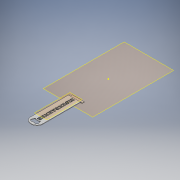
# Autodesk Inventor part: Rost_Heber
Saved by Autodesk Inventor 2018 (Build 220112000, 112)
## iProperties
Created: 2017-10-08
Part Number: Rost_Heber
Material: Generisch
Document SubType Name: Blech
Designer: Jan
Density: 1 g/cm^3
Sheet Metal Rule: Standard_mm
Appearance: Vorgabe
Flat Pattern Width: 4.3 cm
Flat Pattern Length: 17.3098 cm
Flat Pattern Area: 74.432 cm^2
Sheet Metal Width: 43,000 mm
Sheet Metal Length: 173,098 mm
Sheet Metal Area: 7443,205 mm^2
Author: Jan
Autodesk Inventor part; units mm, degrees
ref_plane "YZ Plane" through (0, 0, 0) normal (1, 0, 0) x (0, 1, 0)
ref_plane "XZ Plane" through (0, 0, 0) normal (0, 1, 0) x (-1, 0, 0)
ref_plane "XY Plane" through (0, 0, 0) normal (0, 0, 1) x (1, 0, 0)
ref_plane "Arbeitsebene1" through (0, 0, 0) normal (0, 0, 1) x (1, 0, 0)
sketch "Skizze1" plane through (0, 0, 0) normal (0, 0, 1) x (1, 0, 0)
  arc A0 (31.5, -113.5) -> (26.5, -108.5) centre (26.5, -113.5) ccw
  line L0 (26.5, -108.5) -> (-26.5, -108.5)
  arc A1 (-26.5, -108.5) -> (-31.5, -113.5) centre (-26.5, -113.5) ccw
  line L1 (-31.5, -113.5) -> (-31.5, -124.5)
  line L2 (-31.5, -124.5) -> (-71, -124.5)
  arc A2 (-73, -122.5) -> (-71, -124.5) centre (-71, -122.5) ccw
  line L3 (-73, -122.5) -> (-73, 122.5)
  arc A3 (-71, 124.5) -> (-73, 122.5) centre (-71, 122.5) ccw
  line L4 (-71, 124.5) -> (71, 124.5)
  arc A4 (73, 122.5) -> (71, 124.5) centre (71, 122.5) ccw
  line L5 (73, 122.5) -> (73, -122.5)
  arc A5 (71, -124.5) -> (73, -122.5) centre (71, -122.5) ccw
  line L6 (71, -124.5) -> (31.5, -124.5)
  line L7 (31.5, -124.5) -> (31.5, -113.5)
  line L8 (-22.5, -122.5) -> (-22.5, -117.5)
  line L9 (-22.5, -117.5) -> (22.5, -117.5)
  line L10 (22.5, -117.5) -> (22.5, -122.5)
  line L11 (22.5, -122.5) -> (-22.5, -122.5)
  arc A6 (-81, -122.5) -> (-71, -132.5) centre (-71, -122.5) ccw
  line L12 (71, -132.5) -> (-71, -132.5)
  arc A7 (71, -132.5) -> (81, -122.5) centre (71, -122.5) ccw
  line L13 (81, 122.5) -> (81, -122.5)
  arc A8 (81, 122.5) -> (71, 132.5) centre (71, 122.5) ccw
  line L14 (-71, 132.5) -> (71, 132.5)
  arc A9 (-71, 132.5) -> (-81, 122.5) centre (-71, 122.5) ccw
  line L15 (-81, -122.5) -> (-81, 122.5)
  line L16 (-21.5, -118.5) -> (21.5, -118.5)
  line L17 (21.5, -118.5) -> (21.5, -258.5)
  line L18 (1.5, -278.5) -> (-1.5, -278.5)
  line L19 (-21.5, -258.5) -> (-21.5, -118.5)
  line L20 (-116.2995, 0) -> (116.2995, 0)
  line L21 (0, -314.1009) -> (0, 209.3497)
  arc A10 (-21.5, -258.5) -> (-1.5, -278.5) centre (-1.5, -258.5) ccw
  arc A11 (1.5, -278.5) -> (21.5, -258.5) centre (1.5, -258.5) ccw
  point P0 (0, 0)
  dimension "HeberBreite" = 43
  dimension "d3" = 1
  dimension "HeberLänge" = 160
  dimension "d5" = 20
  measures "HeberBreite" distance of L16.start L16.end
  measures "d3" distance between parallel lines of L9 L16
  measures "HeberLänge" distance between parallel lines of L18 L16
  measures "d5" radius of A10
extrude "Grobblech1" add sketch "Skizze1" along normal blind 2 contours L21 L11 L19 L16 | L16 L17 L11 L21 | L21 L12 L19 L11 | L11 L17 L12 L21 | L21 L18 A10 L19 L12 | L12 L17 A11 L18 L21
sketch "Skizze2" plane through (21.5, -120.5, 2) normal (0, 1, 0) x (-1, 0, 0)
  line L0 (43, 0) -> (0, 0)
  line L1 (0, 0) -> (0, -8.05)
  line L2 (0, -8.05) -> (43, -8.05)
  line L3 (43, -8.05) -> (43, 0)
  constraints: 6 end point, 1 horizontal, 1 perpendicular, 1 vertical
edge flange "Lasche1" height 8.05 angle 90 thickness 2 bend radius 2 thickness toward (0, 1, 0) relief tear relief width 2 relief depth 1 edges at (0, -118.5, 0) wall of the first edge with corners at (-21.5, -120.5, 2) (21.5, -120.5, 2) (21.5, -120.5, -6.05) (-21.5, -120.5, -6.05)
bend "Biegung1"
corner "Ecke1"
sketch "Skizze3" plane through (-21.5, -120.5, -4.05) normal (0, 0, -1) x (-1, 0, 0)
  line L0 (-43, 0) -> (0, 0)
  line L1 (0, 0) -> (0, 12)
  line L2 (0, 12) -> (-43, 12)
  line L3 (-43, 12) -> (-43, 0)
  constraints: 6 end point, 1 horizontal, 1 perpendicular, 1 vertical
edge flange "Lasche2" height 12 angle 90 thickness 2 bend radius 2 thickness toward (0, 0, -1) relief tear relief width 2 relief depth 1 edges at (0, -118.5, -6.05) wall of the first edge with corners at (21.5, -120.5, -4.05) (-21.5, -120.5, -4.05) (-21.5, -108.5, -4.05) (21.5, -108.5, -4.05)
bend "Biegung2"
corner "Ecke2"
sketch "Skizze5" plane through (0, 0, 2) normal (0, 0, 1) x (1, 0, 0)
  line L0 (7, -256.35) -> (7, -254.2861)
  arc A0 (10.3913, -255.0234) -> (7, -254.2861) centre (8.4432, -255.8158) ccw
  line L1 (10.3913, -255.0234) -> (13.6639, -265.2358)
  arc A1 (4.2286, -269.9021) -> (13.6639, -265.2358) centre (7.6833, -265.0153) ccw
  line L2 (21.5, -122.5) -> (-21.5, -122.5) projected
  line L3 (-21.5, -258.5) -> (-21.5, -122.5) projected
  arc A2 (-21.5, -258.5) -> (-1.5, -278.5) centre (-1.5, -258.5) ccw projected
  line L4 (21.5, -122.5) -> (21.5, -258.5) projected
  line L5 (7, -256.35) -> (0, -256.35)
  line L6 (4.2286, -269.9021) -> (0, -269.9021)
  arc A3 (-7, -254.2861) -> (-10.3039, -254.8354) centre (-8.4432, -255.8158) ccw
  line L7 (-10.3039, -254.8354) -> (-13.6607, -265.3108)
  arc A4 (-13.6607, -265.3108) -> (-4.2287, -269.9021) centre (-7.6833, -265.0153) ccw
  line L8 (-7, -256.35) -> (0, -256.35)
  line L9 (-4.2287, -269.9021) -> (0, -269.9021)
  line L10 (-7, -254.2861) -> (-7, -256.35)
  line L11 (0, -312.7) -> (0, 206.7)
  line L12 (1.5, -278.5) -> (-1.5, -278.5) projected
  arc A5 (1.5, -278.5) -> (21.5, -258.5) centre (1.5, -258.5) ccw projected
  constraints: 19 end point, 8 point on circle, 4 centre point, 3 parallel, 2 equal radius, 1 point on line, 1 vertical, 2 other
extrude "Ausklinkung1" cut sketch "Skizze5" against normal blind 2 contours L0 A0 L1 A1 L6 L11 L5 | L11 L9 A4 L7 A3 L10 L8
sketch "Skizze7" plane through (0, 0, 2) normal (0, 0, 1) x (1, 0, 0)
  point P0 (0, 0)
ref_plane "Arbeitsebene2" through (0, 0, 7) normal (0, 0, 1) x (1, 0, 0)
sketch "Skizze8" plane through (0, 0, 7) normal (0, 0, 1) x (1, 0, 0)
  line L0 (5.5899, -125.0888) -> (5.5899, -288.9625) construction
  line L1 (5.5899, -288.9625) -> (-5.6945, -288.9625) construction
  line L2 (-5.6945, -288.9625) -> (-5.6945, -125.0888) construction
  line L3 (-5.6945, -125.0888) -> (5.5899, -125.0888) construction
  line L4 (5.3803, -130.8766) -> (-5.1197, -130.8766)
  line L5 (-5.1197, -130.8766) -> (-5.1197, -126.775)
  line L6 (-5.1197, -126.775) -> (-5.1197, -126.5381)
  spline S0 degree 2 poles (-5.1197, -126.5381) (-5.1197, -126.2008) (-4.9101, -125.8453) (-4.7187, -125.8453) knots 0 0 0 1 2 2 2
  spline S1 degree 2 poles (-4.7187, -125.8453) (-4.4088, -125.8453) (-4.3085, -126.2099) knots 0 0 0 1 1 1
  spline S2 degree 2 poles (-4.3085, -126.2099) (-4.2174, -126.5198) (-4.1809, -126.6201) (-4.108, -126.6748) knots 0 0 0 1 2 2 2
  spline S3 degree 2 poles (-4.108, -126.6748) (-3.9895, -126.7842) (-3.7161, -126.7842) knots 0 0 0 1 1 1
  line L7 (-3.7161, -126.7842) -> (3.9766, -126.7842)
  spline S4 degree 2 poles (3.9766, -126.7842) (4.25, -126.7842) (4.3685, -126.6748) knots 0 0 0 1 1 1
  spline S5 degree 2 poles (4.3685, -126.6748) (4.4415, -126.6201) (4.4779, -126.5198) (4.5599, -126.2099) knots 0 0 0 1 2 2 2
  spline S6 degree 2 poles (4.5599, -126.2099) (4.6602, -125.8453) (4.9792, -125.8453) knots 0 0 0 1 1 1
  spline S7 degree 2 poles (4.9792, -125.8453) (5.1706, -125.8453) (5.3803, -126.2008) (5.3803, -126.5381) knots 0 0 0 1 2 2 2
  line L8 (5.3803, -126.5381) -> (5.3803, -126.775)
  line L9 (5.3803, -126.775) -> (5.3803, -130.8766)
  line L10 (-5.1197, -131.7151) -> (-4.2903, -131.7151)
  spline S8 degree 2 poles (-4.2903, -131.7151) (-4.2174, -132.3167) (-3.9348, -133.1006) (-3.6523, -133.4925) knots 0 0 0 1 2 2 2
  spline S9 degree 2 poles (-3.6523, -133.4925) (-3.3697, -133.8935) (-2.7591, -134.3584) (-2.2578, -134.5771) knots 0 0 0 1 2 2 2
  spline S10 degree 2 poles (-2.2578, -134.5771) (-2.0117, -134.6774) (-1.8385, -134.8961) (-1.8385, -135.0875) knots 0 0 0 1 2 2 2
  spline S11 degree 2 poles (-1.8385, -135.0875) (-1.8385, -135.3519) (-2.0937, -135.5524) (-2.4036, -135.5524) knots 0 0 0 1 2 2 2
  line L11 (-2.4036, -135.5524) -> (-5.1197, -135.5524)
  line L12 (-5.1197, -135.5524) -> (-5.1197, -131.7151)
  line L13 (5.3803, -131.706) -> (5.3803, -135.4248)
  line L14 (5.3803, -135.4248) -> (2.655, -135.4248)
  spline S12 degree 2 poles (2.655, -135.4248) (2.418, -135.4248) (2.2084, -135.206) (2.2084, -134.9599) knots 0 0 0 1 2 2 2
  spline S13 degree 2 poles (2.2084, -134.9599) (2.2084, -134.7594) (2.3451, -134.5771) (2.5639, -134.4951) knots 0 0 0 1 2 2 2
  spline S14 degree 2 poles (2.5639, -134.4951) (3.448, -134.1396) (4.3868, -132.7815) (4.4779, -131.706) knots 0 0 0 1 2 2 2
  line L15 (4.4779, -131.706) -> (5.3803, -131.706)
  line L16 (-0.2252, -131.6605) -> (0.668, -131.6605)
  spline S15 degree 2 poles (0.668, -131.6605) (0.8868, -132.1982) (1.3972, -132.7086) (1.8165, -132.8362) knots 0 0 0 1 2 2 2
  spline S16 degree 2 poles (1.8165, -132.8362) (2.1081, -132.9092) (2.336, -133.1461) (2.336, -133.3649) knots 0 0 0 1 2 2 2
  spline S17 degree 2 poles (2.336, -133.3649) (2.336, -133.6657) (2.1446, -133.775) knots 0 0 0 1 1 1
  spline S18 degree 2 poles (2.1446, -133.775) (2.0443, -133.8388) (1.6889, -133.8388) knots 0 0 0 1 1 1
  line L17 (1.6889, -133.8388) -> (-1.246, -133.8388)
  spline S19 degree 2 poles (-1.246, -133.8388) (-1.6106, -133.8388) (-1.8841, -133.6474) (-1.8841, -133.3831) knots 0 0 0 1 2 2 2
  spline S20 degree 2 poles (-1.8841, -133.3831) (-1.8841, -133.1735) (-1.6653, -132.9365) (-1.4101, -132.8636) knots 0 0 0 1 2 2 2
  spline S21 degree 2 poles (-1.4101, -132.8636) (-0.8815, -132.6995) (-0.3164, -132.1253) (-0.2252, -131.6605) knots 0 0 0 1 2 2 2
  line L18 (-5.1197, -141.9782) -> (-5.1197, -137.8675)
  line L19 (-5.1197, -137.8675) -> (-5.1197, -137.6305)
  spline S22 degree 2 poles (-5.1197, -137.6305) (-5.1197, -137.2933) (-4.9101, -136.9378) (-4.7187, -136.9378) knots 0 0 0 1 2 2 2
  spline S23 degree 2 poles (-4.7187, -136.9378) (-4.4088, -136.9378) (-4.3085, -137.3024) knots 0 0 0 1 1 1
  spline S24 degree 2 poles (-4.3085, -137.3024) (-4.2174, -137.6123) (-4.1809, -137.7125) (-4.108, -137.7672) knots 0 0 0 1 2 2 2
  spline S25 degree 2 poles (-4.108, -137.7672) (-3.9895, -137.8766) (-3.7161, -137.8766) knots 0 0 0 1 1 1
  line L20 (-3.7161, -137.8766) -> (3.9766, -137.8766)
  spline S26 degree 2 poles (3.9766, -137.8766) (4.25, -137.8766) (4.3685, -137.7672) knots 0 0 0 1 1 1
  spline S27 degree 2 poles (4.3685, -137.7672) (4.4415, -137.7125) (4.4779, -137.6123) (4.5599, -137.3024) knots 0 0 0 1 2 2 2
  spline S28 degree 2 poles (4.5599, -137.3024) (4.6602, -136.9378) (4.9792, -136.9378) knots 0 0 0 1 1 1
  spline S29 degree 2 poles (4.9792, -136.9378) (5.1706, -136.9378) (5.3803, -137.2933) (5.3803, -137.6305) knots 0 0 0 1 2 2 2
  line L21 (5.3803, -137.6305) -> (5.3803, -137.8675)
  line L22 (5.3803, -137.8675) -> (5.3803, -141.9782)
  line L23 (5.3803, -141.9782) -> (5.3803, -142.2151)
  spline S30 degree 2 poles (5.3803, -142.2151) (5.3803, -142.5524) (5.1706, -142.9078) (4.9792, -142.9078) knots 0 0 0 1 2 2 2
  spline S31 degree 2 poles (4.9792, -142.9078) (4.6602, -142.9078) (4.5599, -142.5433) knots 0 0 0 1 1 1
  spline S32 degree 2 poles (4.5599, -142.5433) (4.4779, -142.2334) (4.4415, -142.1331) (4.3685, -142.0784) knots 0 0 0 1 2 2 2
  spline S33 degree 2 poles (4.3685, -142.0784) (4.25, -141.969) (3.9766, -141.969) knots 0 0 0 1 1 1
  line L24 (3.9766, -141.969) -> (-3.7161, -141.969)
  spline S34 degree 2 poles (-3.7161, -141.969) (-3.9895, -141.969) (-4.108, -142.0784) knots 0 0 0 1 1 1
  spline S35 degree 2 poles (-4.108, -142.0784) (-4.1809, -142.1331) (-4.2174, -142.2334) (-4.3085, -142.5433) knots 0 0 0 1 2 2 2
  spline S36 degree 2 poles (-4.3085, -142.5433) (-4.4088, -142.9078) (-4.7187, -142.9078) knots 0 0 0 1 1 1
  spline S37 degree 2 poles (-4.7187, -142.9078) (-4.9101, -142.9078) (-5.1197, -142.5524) (-5.1197, -142.2151) knots 0 0 0 1 2 2 2
  line L25 (-5.1197, -142.2151) -> (-5.1197, -141.9782)
  line L26 (5.5899, -148.6865) -> (4.7058, -148.6865)
  spline S38 degree 2 poles (4.7058, -148.6865) (4.5691, -148.1123) (4.0222, -147.5107) (3.6303, -147.5107) knots 0 0 0 1 2 2 2
  spline S39 degree 2 poles (3.6303, -147.5107) (3.2383, -147.5107) (2.6641, -148.012) (2.3998, -148.568) knots 0 0 0 1 2 2 2
  spline S40 degree 2 poles (2.3998, -148.568) (2.2266, -148.9599) (1.7253, -150.3271) knots 0 0 0 1 1 1
  spline S41 degree 2 poles (1.7253, -150.3271) (1.4245, -151.1565) (0.9415, -152.068) (0.5769, -152.4782) knots 0 0 0 1 2 2 2
  spline S42 degree 2 poles (0.5769, -152.4782) (-0.371, -153.5628) (-1.6927, -153.5628) knots 0 0 0 1 1 1
  spline S43 degree 2 poles (-1.6927, -153.5628) (-2.677, -153.5628) (-4.3268, -152.3779) (-4.8007, -151.348) knots 0 0 0 1 2 2 2
  spline S44 degree 2 poles (-4.8007, -151.348) (-5.0468, -150.792) (-5.3294, -149.4795) (-5.3294, -148.9052) knots 0 0 0 1 2 2 2
  line L27 (-5.3294, -148.9052) -> (-4.4544, -148.9052)
  spline S45 degree 2 poles (-4.4544, -148.9052) (-4.2903, -149.7073) (-3.7161, -150.4183) (-3.2239, -150.4183) knots 0 0 0 1 2 2 2
  spline S46 degree 2 poles (-3.2239, -150.4183) (-2.7044, -150.4183) (-2.3124, -149.8623) knots 0 0 0 1 1 1
  spline S47 degree 2 poles (-2.3124, -149.8623) (-2.0572, -149.4977) (-1.6835, -148.4586) knots 0 0 0 1 1 1
  spline S48 degree 2 poles (-1.6835, -148.4586) (-1.2643, -147.3284) (-0.9088, -146.4899) (-0.6718, -146.098) knots 0 0 0 1 2 2 2
  spline S49 degree 2 poles (-0.6718, -146.098) (0.3581, -144.3662) (2.0717, -144.3662) knots 0 0 0 1 1 1
  spline S50 degree 2 poles (2.0717, -144.3662) (2.9467, -144.3662) (4.4323, -145.2321) (4.8881, -146.0068) knots 0 0 0 1 2 2 2
  spline S51 degree 2 poles (4.8881, -146.0068) (5.517, -147.0914) (5.5899, -148.6865) knots 0 0 0 1 1 1
  line L28 (-4.4544, -148.2034) -> (-5.3294, -148.2034)
  spline S52 degree 2 poles (-5.3294, -148.2034) (-5.3294, -147.4469) (-4.9739, -146.5355) knots 0 0 0 1 1 1
  spline S53 degree 2 poles (-4.9739, -146.5355) (-4.8372, -146.1891) (-4.7643, -145.9339) (-4.7643, -145.8154) knots 0 0 0 1 2 2 2
  spline S54 degree 2 poles (-4.7643, -145.8154) (-4.7643, -145.6331) (-4.8645, -145.4417) (-5.0651, -145.2412) knots 0 0 0 1 2 2 2
  spline S55 degree 2 poles (-5.0651, -145.2412) (-5.2291, -145.0771) (-5.2291, -144.8857) knots 0 0 0 1 1 1
  spline S56 degree 2 poles (-5.2291, -144.8857) (-5.2291, -144.3662) (-4.5638, -144.3662) knots 0 0 0 1 1 1
  line L29 (-4.5638, -144.3662) -> (-1.7656, -144.3662)
  spline S57 degree 2 poles (-1.7656, -144.3662) (-1.5559, -144.3662) (-1.2552, -144.6578) (-1.246, -144.8857) knots 0 0 0 1 2 2 2
  spline S58 degree 2 poles (-1.246, -144.8857) (-1.2369, -145.0862) (-1.4466, -145.3141) (-1.7109, -145.3961) knots 0 0 0 1 2 2 2
  spline S59 degree 2 poles (-1.7109, -145.3961) (-2.3671, -145.6149) (-3.5247, -146.417) (-3.9166, -146.9456) knots 0 0 0 1 2 2 2
  spline S60 degree 2 poles (-3.9166, -146.9456) (-4.3359, -147.4925) (-4.4544, -148.2034) knots 0 0 0 1 1 1
  line L30 (4.7058, -149.4157) -> (5.5534, -149.4157)
  spline S61 degree 2 poles (5.5534, -149.4157) (5.517, -149.9716) (5.3347, -150.7828) (5.0704, -151.5302) knots 0 0 0 1 2 2 2
  spline S62 degree 2 poles (5.0704, -151.5302) (5.0066, -151.7125) (5.0066, -151.831) knots 0 0 0 1 1 1
  spline S63 degree 2 poles (5.0066, -151.831) (5.0066, -152.0042) (5.1068, -152.0953) knots 0 0 0 1 1 1
  line L31 (5.1068, -152.0953) -> (5.3347, -152.2959)
  spline S64 degree 2 poles (5.3347, -152.2959) (5.5079, -152.4417) (5.5079, -152.6513) knots 0 0 0 1 1 1
  spline S65 degree 2 poles (5.5079, -152.6513) (5.5079, -152.9065) (5.2071, -153.1344) (4.8881, -153.1344) knots 0 0 0 1 2 2 2
  line L32 (4.8881, -153.1344) -> (2.3451, -153.1344)
  spline S66 degree 2 poles (2.3451, -153.1344) (2.1172, -153.1344) (1.8347, -152.8336) (1.8347, -152.5875) knots 0 0 0 1 2 2 2
  spline S67 degree 2 poles (1.8347, -152.5875) (1.8347, -152.4052) (1.9349, -152.2503) knots 0 0 0 1 1 1
  spline S68 degree 2 poles (1.9349, -152.2503) (1.9987, -152.1683) (2.1719, -152.068) (2.3816, -152.0224) knots 0 0 0 1 2 2 2
  spline S69 degree 2 poles (2.3816, -152.0224) (2.7644, -151.9131) (3.5573, -151.4209) (3.8764, -151.0836) knots 0 0 0 1 2 2 2
  spline S70 degree 2 poles (3.8764, -151.0836) (4.5053, -150.4183) (4.7058, -149.4157) knots 0 0 0 1 1 1
  line L33 (5.3803, -160.0433) -> (-5.1197, -160.0433)
  line L34 (-5.1197, -160.0433) -> (-5.1197, -155.9417)
  line L35 (-5.1197, -155.9417) -> (-5.1197, -155.7047)
  spline S71 degree 2 poles (-5.1197, -155.7047) (-5.1197, -155.3675) (-4.9101, -155.012) (-4.7187, -155.012) knots 0 0 0 1 2 2 2
  spline S72 degree 2 poles (-4.7187, -155.012) (-4.4088, -155.012) (-4.3085, -155.3766) knots 0 0 0 1 1 1
  spline S73 degree 2 poles (-4.3085, -155.3766) (-4.2174, -155.6865) (-4.1809, -155.7868) (-4.108, -155.8414) knots 0 0 0 1 2 2 2
  spline S74 degree 2 poles (-4.108, -155.8414) (-3.9895, -155.9508) (-3.7161, -155.9508) knots 0 0 0 1 1 1
  line L36 (-3.7161, -155.9508) -> (3.9766, -155.9508)
  spline S75 degree 2 poles (3.9766, -155.9508) (4.25, -155.9508) (4.3685, -155.8414) knots 0 0 0 1 1 1
  spline S76 degree 2 poles (4.3685, -155.8414) (4.4415, -155.7868) (4.4779, -155.6865) (4.5599, -155.3766) knots 0 0 0 1 2 2 2
  spline S77 degree 2 poles (4.5599, -155.3766) (4.6602, -155.012) (4.9792, -155.012) knots 0 0 0 1 1 1
  spline S78 degree 2 poles (4.9792, -155.012) (5.1706, -155.012) (5.3803, -155.3675) (5.3803, -155.7047) knots 0 0 0 1 2 2 2
  line L37 (5.3803, -155.7047) -> (5.3803, -155.9417)
  line L38 (5.3803, -155.9417) -> (5.3803, -160.0433)
  line L39 (-5.1197, -160.8818) -> (-4.2903, -160.8818)
  spline S79 degree 2 poles (-4.2903, -160.8818) (-4.2174, -161.4834) (-3.9348, -162.2672) (-3.6523, -162.6591) knots 0 0 0 1 2 2 2
  spline S80 degree 2 poles (-3.6523, -162.6591) (-3.3697, -163.0602) (-2.7591, -163.525) (-2.2578, -163.7438) knots 0 0 0 1 2 2 2
  spline S81 degree 2 poles (-2.2578, -163.7438) (-2.0117, -163.844) (-1.8385, -164.0628) (-1.8385, -164.2542) knots 0 0 0 1 2 2 2
  spline S82 degree 2 poles (-1.8385, -164.2542) (-1.8385, -164.5185) (-2.0937, -164.719) (-2.4036, -164.719) knots 0 0 0 1 2 2 2
  line L40 (-2.4036, -164.719) -> (-5.1197, -164.719)
  line L41 (-5.1197, -164.719) -> (-5.1197, -160.8818)
  line L42 (5.3803, -160.8727) -> (5.3803, -164.5914)
  line L43 (5.3803, -164.5914) -> (2.655, -164.5914)
  spline S83 degree 2 poles (2.655, -164.5914) (2.418, -164.5914) (2.2084, -164.3727) (2.2084, -164.1266) knots 0 0 0 1 2 2 2
  spline S84 degree 2 poles (2.2084, -164.1266) (2.2084, -163.9261) (2.3451, -163.7438) (2.5639, -163.6618) knots 0 0 0 1 2 2 2
  spline S85 degree 2 poles (2.5639, -163.6618) (3.448, -163.3063) (4.3868, -161.9482) (4.4779, -160.8727) knots 0 0 0 1 2 2 2
  line L44 (4.4779, -160.8727) -> (5.3803, -160.8727)
  line L45 (-0.2252, -160.8271) -> (0.668, -160.8271)
  spline S86 degree 2 poles (0.668, -160.8271) (0.8868, -161.3649) (1.3972, -161.8753) (1.8165, -162.0029) knots 0 0 0 1 2 2 2
  spline S87 degree 2 poles (1.8165, -162.0029) (2.1081, -162.0758) (2.336, -162.3128) (2.336, -162.5315) knots 0 0 0 1 2 2 2
  spline S88 degree 2 poles (2.336, -162.5315) (2.336, -162.8323) (2.1446, -162.9417) knots 0 0 0 1 1 1
  spline S89 degree 2 poles (2.1446, -162.9417) (2.0443, -163.0055) (1.6889, -163.0055) knots 0 0 0 1 1 1
  line L46 (1.6889, -163.0055) -> (-1.246, -163.0055)
  spline S90 degree 2 poles (-1.246, -163.0055) (-1.6106, -163.0055) (-1.8841, -162.8141) (-1.8841, -162.5498) knots 0 0 0 1 2 2 2
  spline S91 degree 2 poles (-1.8841, -162.5498) (-1.8841, -162.3401) (-1.6653, -162.1032) (-1.4101, -162.0302) knots 0 0 0 1 2 2 2
  spline S92 degree 2 poles (-1.4101, -162.0302) (-0.8815, -161.8662) (-0.3164, -161.292) (-0.2252, -160.8271) knots 0 0 0 1 2 2 2
  line L47 (5.3803, -171.3271) -> (-1.7291, -176.2308)
  line L48 (-1.7291, -176.2308) -> (-5.1197, -176.2308)
  line L49 (-5.1197, -176.2308) -> (-5.1197, -173.7151)
  line L50 (-5.1197, -173.7151) -> (3.8764, -167.4534)
  spline S93 degree 2 poles (3.8764, -167.4534) (4.1771, -167.2438) (4.405, -166.9886) (4.4597, -166.7881) knots 0 0 0 1 2 2 2
  line L51 (4.4597, -166.7881) -> (4.5691, -166.4326)
  spline S94 degree 2 poles (4.5691, -166.4326) (4.6055, -166.2959) (4.806, -166.1318) (4.9245, -166.1318) knots 0 0 0 1 2 2 2
  spline S95 degree 2 poles (4.9245, -166.1318) (5.0612, -166.1318) (5.28, -166.2959) (5.3256, -166.4326) knots 0 0 0 1 2 2 2
  spline S96 degree 2 poles (5.3256, -166.4326) (5.3803, -166.5875) (5.3803, -167.2802) knots 0 0 0 1 1 1
  line L52 (5.3803, -167.2802) -> (5.3803, -171.3271)
  line L53 (2.6732, -167.4625) -> (1.3243, -168.4378)
  line L54 (1.3243, -168.4378) -> (-2.7955, -168.4378)
  spline S97 degree 2 poles (-2.7955, -168.4378) (-3.3333, -168.4378) (-4.026, -168.8753) (-4.2539, -169.3401) knots 0 0 0 1 2 2 2
  line L55 (-4.2539, -169.3401) -> (-4.3815, -169.6227)
  spline S98 degree 2 poles (-4.3815, -169.6227) (-4.4999, -169.8597) (-4.7278, -169.8597) knots 0 0 0 1 1 1
  spline S99 degree 2 poles (-4.7278, -169.8597) (-4.901, -169.8597) (-5.0195, -169.6865) knots 0 0 0 1 1 1
  spline S100 degree 2 poles (-5.0195, -169.6865) (-5.1197, -169.5407) (-5.1197, -169.0758) knots 0 0 0 1 1 1
  line L56 (-5.1197, -169.0758) -> (-5.1197, -166.943)
  spline S101 degree 2 poles (-5.1197, -166.943) (-5.1197, -166.1045) (-4.7187, -166.1045) knots 0 0 0 1 1 1
  spline S102 degree 2 poles (-4.7187, -166.1045) (-4.582, -166.1045) (-4.4179, -166.2776) (-4.2812, -166.5784) knots 0 0 0 1 2 2 2
  spline S103 degree 2 poles (-4.2812, -166.5784) (-3.871, -167.4625) (-2.7955, -167.4625) knots 0 0 0 1 1 1
  line L57 (-2.7955, -167.4625) -> (2.6732, -167.4625)
  line L58 (-0.4986, -176.2308) -> (0.8777, -175.2555)
  line L59 (0.8777, -175.2555) -> (3.0105, -175.2555)
  spline S104 degree 2 poles (3.0105, -175.2555) (3.6576, -175.2555) (4.3412, -174.7998) (4.5873, -174.2347) knots 0 0 0 1 2 2 2
  spline S105 degree 2 poles (4.5873, -174.2347) (4.6602, -174.0341) (4.8425, -173.8883) (4.9792, -173.8883) knots 0 0 0 1 2 2 2
  spline S106 degree 2 poles (4.9792, -173.8883) (5.1889, -173.8883) (5.3803, -174.2164) (5.3803, -174.5719) knots 0 0 0 1 2 2 2
  line L60 (5.3803, -174.5719) -> (5.3803, -176.8779)
  spline S107 degree 2 poles (5.3803, -176.8779) (5.3803, -177.3519) (5.2527, -177.4977) knots 0 0 0 1 1 1
  spline S108 degree 2 poles (5.2527, -177.4977) (5.1342, -177.6526) (4.961, -177.6526) knots 0 0 0 1 1 1
  spline S109 degree 2 poles (4.961, -177.6526) (4.806, -177.6526) (4.642, -177.4795) (4.5053, -177.1422) knots 0 0 0 1 2 2 2
  spline S110 degree 2 poles (4.5053, -177.1422) (4.2956, -176.6591) (3.8672, -176.4039) knots 0 0 0 1 1 1
  spline S111 degree 2 poles (3.8672, -176.4039) (3.5482, -176.2308) (3.0105, -176.2308) knots 0 0 0 1 1 1
  line L61 (3.0105, -176.2308) -> (-0.4986, -176.2308)
  line L62 (5.3803, -183.8232) -> (-5.1197, -183.8232)
  line L63 (-5.1197, -183.8232) -> (-5.1197, -179.7216)
  line L64 (-5.1197, -179.7216) -> (-5.1197, -179.4847)
  spline S112 degree 2 poles (-5.1197, -179.4847) (-5.1197, -179.1474) (-4.9101, -178.792) (-4.7187, -178.792) knots 0 0 0 1 2 2 2
  spline S113 degree 2 poles (-4.7187, -178.792) (-4.4088, -178.792) (-4.3085, -179.1565) knots 0 0 0 1 1 1
  spline S114 degree 2 poles (-4.3085, -179.1565) (-4.2174, -179.4664) (-4.1809, -179.5667) (-4.108, -179.6214) knots 0 0 0 1 2 2 2
  spline S115 degree 2 poles (-4.108, -179.6214) (-3.9895, -179.7308) (-3.7161, -179.7308) knots 0 0 0 1 1 1
  line L65 (-3.7161, -179.7308) -> (3.9766, -179.7308)
  spline S116 degree 2 poles (3.9766, -179.7308) (4.25, -179.7308) (4.3685, -179.6214) knots 0 0 0 1 1 1
  spline S117 degree 2 poles (4.3685, -179.6214) (4.4415, -179.5667) (4.4779, -179.4664) (4.5599, -179.1565) knots 0 0 0 1 2 2 2
  spline S118 degree 2 poles (4.5599, -179.1565) (4.6602, -178.792) (4.9792, -178.792) knots 0 0 0 1 1 1
  spline S119 degree 2 poles (4.9792, -178.792) (5.1706, -178.792) (5.3803, -179.1474) (5.3803, -179.4847) knots 0 0 0 1 2 2 2
  line L66 (5.3803, -179.4847) -> (5.3803, -179.7216)
  line L67 (5.3803, -179.7216) -> (5.3803, -183.8232)
  spline S120 degree 2 poles (0.3125, -186.6943) (0.1758, -187.5237) (-0.0794, -188.4261) (-0.2799, -188.7815) knots 0 0 0 1 2 2 2
  spline S121 degree 2 poles (-0.2799, -188.7815) (-0.6171, -189.4013) (-1.7018, -190.0576) (-2.3671, -190.0576) knots 0 0 0 1 2 2 2
  spline S122 degree 2 poles (-2.3671, -190.0576) (-3.6796, -190.0576) (-4.4179, -188.8909) knots 0 0 0 1 1 1
  spline S123 degree 2 poles (-4.4179, -188.8909) (-4.8007, -188.2985) (-5.1197, -186.8493) (-5.1197, -185.6735) knots 0 0 0 1 2 2 2
  line L68 (-5.1197, -185.6735) -> (-5.1197, -184.5706)
  line L69 (-5.1197, -184.5706) -> (-4.3085, -184.5706)
  spline S124 degree 2 poles (-4.3085, -184.5706) (-4.2903, -184.9443) (-4.1627, -185.3636) (-4.0078, -185.5368) knots 0 0 0 1 2 2 2
  spline S125 degree 2 poles (-4.0078, -185.5368) (-3.7161, -185.8375) (-3.1236, -185.8375) knots 0 0 0 1 1 1
  line L70 (-3.1236, -185.8375) -> (-1.3736, -185.8375)
  spline S126 degree 2 poles (-1.3736, -185.8375) (-0.9908, -185.8375) (-0.5624, -185.6826) (-0.3802, -185.473) knots 0 0 0 1 2 2 2
  spline S127 degree 2 poles (-0.3802, -185.473) (-0.2434, -185.318) (-0.1249, -184.9443) (-0.0794, -184.6071) knots 0 0 0 1 2 2 2
  line L71 (-0.0794, -184.6071) -> (0.7136, -184.6071)
  spline S128 degree 2 poles (0.7136, -184.6071) (0.7409, -184.9443) (0.8503, -185.3271) (0.9688, -185.4821) knots 0 0 0 1 2 2 2
  spline S129 degree 2 poles (0.9688, -185.4821) (1.0873, -185.6279) (1.4519, -185.8284) (1.6068, -185.8375) knots 0 0 0 1 2 2 2
  line L72 (1.6068, -185.8375) -> (2.0352, -185.8375)
  line L73 (2.0352, -185.8375) -> (3.3659, -185.8375)
  spline S130 degree 2 poles (3.3659, -185.8375) (3.5756, -185.8375) (4.0313, -185.6735) (4.1589, -185.555) knots 0 0 0 1 2 2 2
  spline S131 degree 2 poles (4.1589, -185.555) (4.3321, -185.3727) (4.5053, -184.9443) (4.5326, -184.5706) knots 0 0 0 1 2 2 2
  line L74 (4.5326, -184.5706) -> (5.3803, -184.5706)
  line L75 (5.3803, -184.5706) -> (5.3803, -185.637)
  spline S132 degree 2 poles (5.3803, -185.637) (5.3803, -187.7425) (4.6602, -188.8453) knots 0 0 0 1 1 1
  spline S133 degree 2 poles (4.6602, -188.8453) (4.323, -189.3558) (3.3842, -189.8935) (2.8373, -189.8935) knots 0 0 0 1 2 2 2
  spline S134 degree 2 poles (2.8373, -189.8935) (2.2995, -189.8935) (1.3516, -189.3466) (1.0326, -188.8545) knots 0 0 0 1 2 2 2
  spline S135 degree 2 poles (1.0326, -188.8545) (0.7865, -188.499) (0.4766, -187.5602) (0.3125, -186.6943) knots 0 0 0 1 2 2 2
  line L76 (5.3803, -195.1435) -> (5.3803, -198.8623)
  line L77 (5.3803, -198.8623) -> (-3.6614, -201.4235)
  spline S136 degree 2 poles (-3.6614, -201.4235) (-3.8984, -201.4964) (-4.0807, -201.5875) knots 0 0 0 1 1 1
  spline S137 degree 2 poles (-4.0807, -201.5875) (-4.2265, -201.6696) (-4.3177, -201.9612) knots 0 0 0 1 1 1
  spline S138 degree 2 poles (-4.3177, -201.9612) (-4.4088, -202.1982) (-4.5729, -202.3805) (-4.7187, -202.3805) knots 0 0 0 1 2 2 2
  spline S139 degree 2 poles (-4.7187, -202.3805) (-5.1197, -202.3805) (-5.1197, -201.6696) knots 0 0 0 1 1 1
  line L78 (-5.1197, -201.6696) -> (-5.1197, -197.0576)
  spline S140 degree 2 poles (-5.1197, -197.0576) (-5.1197, -196.7841) (-4.8919, -196.456) (-4.7096, -196.456) knots 0 0 0 1 2 2 2
  spline S141 degree 2 poles (-4.7096, -196.456) (-4.5546, -196.456) (-4.3997, -196.6019) (-4.2903, -196.8662) knots 0 0 0 1 2 2 2
  spline S142 degree 2 poles (-4.2903, -196.8662) (-4.2083, -197.0485) (-4.026, -197.1943) (-3.8893, -197.1943) knots 0 0 0 1 2 2 2
  spline S143 degree 2 poles (-3.8893, -197.1943) (-3.7526, -197.1943) (-3.6523, -197.167) knots 0 0 0 1 1 1
  line L79 (-3.6523, -197.167) -> (-2.5403, -196.8662)
  line L80 (-2.5403, -196.8662) -> (-2.5403, -194.2959)
  line L81 (-2.5403, -194.2959) -> (-1.6289, -194.542)
  line L82 (-1.6289, -194.542) -> (-1.6289, -196.611)
  line L83 (-1.6289, -196.611) -> (4.6237, -194.9157)
  line L84 (4.6237, -194.9157) -> (5.3803, -195.1435)
  line L85 (3.4206, -194.5055) -> (1.8347, -194.9795)
  line L86 (1.8347, -194.9795) -> (-3.1328, -193.3388)
  spline S144 degree 2 poles (-3.1328, -193.3388) (-3.3515, -193.2659) (-3.5338, -193.2659) knots 0 0 0 1 1 1
  spline S145 degree 2 poles (-3.5338, -193.2659) (-4.0169, -193.2659) (-4.2265, -193.8128) knots 0 0 0 1 1 1
  line L87 (-4.2265, -193.8128) -> (-4.3541, -194.1318)
  spline S146 degree 2 poles (-4.3541, -194.1318) (-4.4635, -194.4417) (-4.7369, -194.4417) knots 0 0 0 1 1 1
  spline S147 degree 2 poles (-4.7369, -194.4417) (-5.1197, -194.4417) (-5.1197, -193.7672) knots 0 0 0 1 1 1
  line L88 (-5.1197, -193.7672) -> (-5.1197, -191.4248)
  spline S148 degree 2 poles (-5.1197, -191.4248) (-5.1197, -191.0875) (-4.8828, -190.6865) (-4.6731, -190.6865) knots 0 0 0 1 2 2 2
  spline S149 degree 2 poles (-4.6731, -190.6865) (-4.4544, -190.6865) (-4.3085, -191.0966) knots 0 0 0 1 1 1
  spline S150 degree 2 poles (-4.3085, -191.0966) (-4.1627, -191.4703) (-3.944, -191.8349) (-3.7526, -191.999) knots 0 0 0 1 2 2 2
  spline S151 degree 2 poles (-3.7526, -191.999) (-3.4335, -192.2542) (-2.914, -192.4183) knots 0 0 0 1 1 1
  line L89 (-2.914, -192.4183) -> (3.4206, -194.5055)
  line L90 (0.6224, -209.1618) -> (0.6224, -210.6657)
  line L91 (0.6224, -210.6657) -> (3.9766, -210.6657)
  spline S152 degree 2 poles (3.9766, -210.6657) (4.4141, -210.6657) (4.487, -210.4013) knots 0 0 0 1 1 1
  line L92 (4.487, -210.4013) -> (4.5599, -210.1006)
  spline S153 degree 2 poles (4.5599, -210.1006) (4.6602, -209.7542) (4.9792, -209.7542) knots 0 0 0 1 1 1
  spline S154 degree 2 poles (4.9792, -209.7542) (5.3803, -209.7542) (5.3803, -210.4196) knots 0 0 0 1 1 1
  line L93 (5.3803, -210.4196) -> (5.3803, -210.6565)
  line L94 (5.3803, -210.6565) -> (5.3803, -214.7581)
  line L95 (5.3803, -214.7581) -> (5.3803, -215.0042)
  spline S155 degree 2 poles (5.3803, -215.0042) (5.3803, -215.6969) (4.9792, -215.6969) knots 0 0 0 1 1 1
  spline S156 degree 2 poles (4.9792, -215.6969) (4.6602, -215.6969) (4.5599, -215.3323) knots 0 0 0 1 1 1
  spline S157 degree 2 poles (4.5599, -215.3323) (4.4779, -215.0224) (4.4415, -214.9222) (4.3685, -214.8675) knots 0 0 0 1 2 2 2
  spline S158 degree 2 poles (4.3685, -214.8675) (4.25, -214.7581) (3.9766, -214.7581) knots 0 0 0 1 1 1
  line L96 (3.9766, -214.7581) -> (-3.6888, -214.7581)
  spline S159 degree 2 poles (-3.6888, -214.7581) (-4.1171, -214.7581) (-4.2083, -215.0315) knots 0 0 0 1 1 1
  line L97 (-4.2083, -215.0315) -> (-4.2903, -215.3323)
  spline S160 degree 2 poles (-4.2903, -215.3323) (-4.3906, -215.6969) (-4.7096, -215.6969) knots 0 0 0 1 1 1
  spline S161 degree 2 poles (-4.7096, -215.6969) (-5.1197, -215.6969) (-5.1197, -215.0042) knots 0 0 0 1 1 1
  line L98 (-5.1197, -215.0042) -> (-5.1197, -214.7581)
  line L99 (-5.1197, -214.7581) -> (-5.1197, -210.6565)
  line L100 (-5.1197, -210.6565) -> (-5.1197, -210.4013)
  spline S162 degree 2 poles (-5.1197, -210.4013) (-5.1197, -209.7542) (-4.7096, -209.7542) knots 0 0 0 1 1 1
  spline S163 degree 2 poles (-4.7096, -209.7542) (-4.3906, -209.7542) (-4.2903, -210.1006) knots 0 0 0 1 1 1
  line L101 (-4.2903, -210.1006) -> (-4.2083, -210.4013)
  spline S164 degree 2 poles (-4.2083, -210.4013) (-4.1354, -210.6657) (-3.6888, -210.6657) knots 0 0 0 1 1 1
  line L102 (-3.6888, -210.6657) -> (-0.1432, -210.6657)
  line L103 (-0.1432, -210.6657) -> (-0.1432, -209.1618)
  line L104 (-0.1432, -209.1618) -> (0.6224, -209.1618)
  line L105 (-5.1197, -208.387) -> (-5.1197, -204.2763)
  line L106 (-5.1197, -204.2763) -> (-5.1197, -204.0394)
  spline S165 degree 2 poles (-5.1197, -204.0394) (-5.1197, -203.7021) (-4.9101, -203.3466) (-4.7187, -203.3466) knots 0 0 0 1 2 2 2
  spline S166 degree 2 poles (-4.7187, -203.3466) (-4.4088, -203.3466) (-4.3085, -203.7112) knots 0 0 0 1 1 1
  spline S167 degree 2 poles (-4.3085, -203.7112) (-4.2174, -204.0211) (-4.1809, -204.1214) (-4.108, -204.1761) knots 0 0 0 1 2 2 2
  spline S168 degree 2 poles (-4.108, -204.1761) (-3.9895, -204.2854) (-3.7161, -204.2854) knots 0 0 0 1 1 1
  line L107 (-3.7161, -204.2854) -> (3.9766, -204.2854)
  spline S169 degree 2 poles (3.9766, -204.2854) (4.25, -204.2854) (4.3685, -204.1761) knots 0 0 0 1 1 1
  spline S170 degree 2 poles (4.3685, -204.1761) (4.4415, -204.1214) (4.4779, -204.0211) (4.5599, -203.7112) knots 0 0 0 1 2 2 2
  spline S171 degree 2 poles (4.5599, -203.7112) (4.6602, -203.3466) (4.9792, -203.3466) knots 0 0 0 1 1 1
  spline S172 degree 2 poles (4.9792, -203.3466) (5.1706, -203.3466) (5.3803, -203.7021) (5.3803, -204.0394) knots 0 0 0 1 2 2 2
  line L108 (5.3803, -204.0394) -> (5.3803, -204.2763)
  line L109 (5.3803, -204.2763) -> (5.3803, -208.387)
  line L110 (5.3803, -208.387) -> (5.3803, -208.624)
  spline S173 degree 2 poles (5.3803, -208.624) (5.3803, -209.2802) (4.9792, -209.2802) knots 0 0 0 1 1 1
  spline S174 degree 2 poles (4.9792, -209.2802) (4.6602, -209.2802) (4.5599, -208.9339) knots 0 0 0 1 1 1
  line L111 (4.5599, -208.9339) -> (4.487, -208.6422)
  spline S175 degree 2 poles (4.487, -208.6422) (4.4141, -208.3779) (3.9766, -208.3779) knots 0 0 0 1 1 1
  line L112 (3.9766, -208.3779) -> (-3.7161, -208.3779)
  spline S176 degree 2 poles (-3.7161, -208.3779) (-4.1536, -208.3779) (-4.2265, -208.6422) knots 0 0 0 1 1 1
  line L113 (-4.2265, -208.6422) -> (-4.3085, -208.9339)
  spline S177 degree 2 poles (-4.3085, -208.9339) (-4.3997, -209.2802) (-4.7187, -209.2802) knots 0 0 0 1 1 1
  spline S178 degree 2 poles (-4.7187, -209.2802) (-5.1197, -209.2802) (-5.1197, -208.624) knots 0 0 0 1 1 1
  line L114 (-5.1197, -208.624) -> (-5.1197, -208.387)
  line L115 (5.3803, -222.6331) -> (-1.7291, -227.5368)
  line L116 (-1.7291, -227.5368) -> (-5.1197, -227.5368)
  line L117 (-5.1197, -227.5368) -> (-5.1197, -225.0211)
  line L118 (-5.1197, -225.0211) -> (3.8764, -218.7594)
  spline S179 degree 2 poles (3.8764, -218.7594) (4.1771, -218.5498) (4.405, -218.2946) (4.4597, -218.094) knots 0 0 0 1 2 2 2
  line L119 (4.4597, -218.094) -> (4.5691, -217.7386)
  spline S180 degree 2 poles (4.5691, -217.7386) (4.6055, -217.6019) (4.806, -217.4378) (4.9245, -217.4378) knots 0 0 0 1 2 2 2
  spline S181 degree 2 poles (4.9245, -217.4378) (5.0612, -217.4378) (5.28, -217.6019) (5.3256, -217.7386) knots 0 0 0 1 2 2 2
  spline S182 degree 2 poles (5.3256, -217.7386) (5.3803, -217.8935) (5.3803, -218.5862) knots 0 0 0 1 1 1
  line L120 (5.3803, -218.5862) -> (5.3803, -222.6331)
  line L121 (2.6732, -218.7685) -> (1.3243, -219.7438)
  line L122 (1.3243, -219.7438) -> (-2.7955, -219.7438)
  spline S183 degree 2 poles (-2.7955, -219.7438) (-3.3333, -219.7438) (-4.026, -220.1813) (-4.2539, -220.6461) knots 0 0 0 1 2 2 2
  line L123 (-4.2539, -220.6461) -> (-4.3815, -220.9287)
  spline S184 degree 2 poles (-4.3815, -220.9287) (-4.4999, -221.1657) (-4.7278, -221.1657) knots 0 0 0 1 1 1
  spline S185 degree 2 poles (-4.7278, -221.1657) (-4.901, -221.1657) (-5.0195, -220.9925) knots 0 0 0 1 1 1
  spline S186 degree 2 poles (-5.0195, -220.9925) (-5.1197, -220.8466) (-5.1197, -220.3818) knots 0 0 0 1 1 1
  line L124 (-5.1197, -220.3818) -> (-5.1197, -218.249)
  spline S187 degree 2 poles (-5.1197, -218.249) (-5.1197, -217.4104) (-4.7187, -217.4104) knots 0 0 0 1 1 1
  spline S188 degree 2 poles (-4.7187, -217.4104) (-4.582, -217.4104) (-4.4179, -217.5836) (-4.2812, -217.8844) knots 0 0 0 1 2 2 2
  spline S189 degree 2 poles (-4.2812, -217.8844) (-3.871, -218.7685) (-2.7955, -218.7685) knots 0 0 0 1 1 1
  line L125 (-2.7955, -218.7685) -> (2.6732, -218.7685)
  line L126 (-0.4986, -227.5368) -> (0.8777, -226.5615)
  line L127 (0.8777, -226.5615) -> (3.0105, -226.5615)
  spline S190 degree 2 poles (3.0105, -226.5615) (3.6576, -226.5615) (4.3412, -226.1058) (4.5873, -225.5407) knots 0 0 0 1 2 2 2
  spline S191 degree 2 poles (4.5873, -225.5407) (4.6602, -225.3401) (4.8425, -225.1943) (4.9792, -225.1943) knots 0 0 0 1 2 2 2
  spline S192 degree 2 poles (4.9792, -225.1943) (5.1889, -225.1943) (5.3803, -225.5224) (5.3803, -225.8779) knots 0 0 0 1 2 2 2
  line L128 (5.3803, -225.8779) -> (5.3803, -228.1839)
  spline S193 degree 2 poles (5.3803, -228.1839) (5.3803, -228.6578) (5.2527, -228.8037) knots 0 0 0 1 1 1
  spline S194 degree 2 poles (5.2527, -228.8037) (5.1342, -228.9586) (4.961, -228.9586) knots 0 0 0 1 1 1
  spline S195 degree 2 poles (4.961, -228.9586) (4.806, -228.9586) (4.642, -228.7854) (4.5053, -228.4482) knots 0 0 0 1 2 2 2
  spline S196 degree 2 poles (4.5053, -228.4482) (4.2956, -227.9651) (3.8672, -227.7099) knots 0 0 0 1 1 1
  spline S197 degree 2 poles (3.8672, -227.7099) (3.5482, -227.5368) (3.0105, -227.5368) knots 0 0 0 1 1 1
  line L129 (3.0105, -227.5368) -> (-0.4986, -227.5368)
  line L130 (5.3803, -235.1292) -> (-5.1197, -235.1292)
  line L131 (-5.1197, -235.1292) -> (-5.1197, -231.0276)
  line L132 (-5.1197, -231.0276) -> (-5.1197, -230.7907)
  spline S198 degree 2 poles (-5.1197, -230.7907) (-5.1197, -230.4534) (-4.9101, -230.0979) (-4.7187, -230.0979) knots 0 0 0 1 2 2 2
  spline S199 degree 2 poles (-4.7187, -230.0979) (-4.4088, -230.0979) (-4.3085, -230.4625) knots 0 0 0 1 1 1
  spline S200 degree 2 poles (-4.3085, -230.4625) (-4.2174, -230.7724) (-4.1809, -230.8727) (-4.108, -230.9274) knots 0 0 0 1 2 2 2
  spline S201 degree 2 poles (-4.108, -230.9274) (-3.9895, -231.0368) (-3.7161, -231.0368) knots 0 0 0 1 1 1
  line L133 (-3.7161, -231.0368) -> (3.9766, -231.0368)
  spline S202 degree 2 poles (3.9766, -231.0368) (4.25, -231.0368) (4.3685, -230.9274) knots 0 0 0 1 1 1
  spline S203 degree 2 poles (4.3685, -230.9274) (4.4415, -230.8727) (4.4779, -230.7724) (4.5599, -230.4625) knots 0 0 0 1 2 2 2
  spline S204 degree 2 poles (4.5599, -230.4625) (4.6602, -230.0979) (4.9792, -230.0979) knots 0 0 0 1 1 1
  spline S205 degree 2 poles (4.9792, -230.0979) (5.1706, -230.0979) (5.3803, -230.4534) (5.3803, -230.7907) knots 0 0 0 1 2 2 2
  line L134 (5.3803, -230.7907) -> (5.3803, -231.0276)
  line L135 (5.3803, -231.0276) -> (5.3803, -235.1292)
  line L136 (-5.1197, -235.9677) -> (-4.2903, -235.9677)
  spline S206 degree 2 poles (-4.2903, -235.9677) (-4.2174, -236.5693) (-3.9348, -237.3532) (-3.6523, -237.7451) knots 0 0 0 1 2 2 2
  spline S207 degree 2 poles (-3.6523, -237.7451) (-3.3697, -238.1461) (-2.7591, -238.611) (-2.2578, -238.8297) knots 0 0 0 1 2 2 2
  spline S208 degree 2 poles (-2.2578, -238.8297) (-2.0117, -238.93) (-1.8385, -239.1487) (-1.8385, -239.3401) knots 0 0 0 1 2 2 2
  spline S209 degree 2 poles (-1.8385, -239.3401) (-1.8385, -239.6045) (-2.0937, -239.805) (-2.4036, -239.805) knots 0 0 0 1 2 2 2
  line L137 (-2.4036, -239.805) -> (-5.1197, -239.805)
  line L138 (-5.1197, -239.805) -> (-5.1197, -235.9677)
  line L139 (5.3803, -235.9586) -> (5.3803, -239.6774)
  line L140 (5.3803, -239.6774) -> (2.655, -239.6774)
  spline S210 degree 2 poles (2.655, -239.6774) (2.418, -239.6774) (2.2084, -239.4586) (2.2084, -239.2125) knots 0 0 0 1 2 2 2
  spline S211 degree 2 poles (2.2084, -239.2125) (2.2084, -239.012) (2.3451, -238.8297) (2.5639, -238.7477) knots 0 0 0 1 2 2 2
  spline S212 degree 2 poles (2.5639, -238.7477) (3.448, -238.3922) (4.3868, -237.0341) (4.4779, -235.9586) knots 0 0 0 1 2 2 2
  line L141 (4.4779, -235.9586) -> (5.3803, -235.9586)
  line L142 (-0.2252, -235.9131) -> (0.668, -235.9131)
  spline S213 degree 2 poles (0.668, -235.9131) (0.8868, -236.4508) (1.3972, -236.9612) (1.8165, -237.0888) knots 0 0 0 1 2 2 2
  spline S214 degree 2 poles (1.8165, -237.0888) (2.1081, -237.1618) (2.336, -237.3987) (2.336, -237.6175) knots 0 0 0 1 2 2 2
  spline S215 degree 2 poles (2.336, -237.6175) (2.336, -237.9183) (2.1446, -238.0276) knots 0 0 0 1 1 1
  spline S216 degree 2 poles (2.1446, -238.0276) (2.0443, -238.0914) (1.6889, -238.0914) knots 0 0 0 1 1 1
  line L143 (1.6889, -238.0914) -> (-1.246, -238.0914)
  spline S217 degree 2 poles (-1.246, -238.0914) (-1.6106, -238.0914) (-1.8841, -237.9) (-1.8841, -237.6357) knots 0 0 0 1 2 2 2
  spline S218 degree 2 poles (-1.8841, -237.6357) (-1.8841, -237.4261) (-1.6653, -237.1891) (-1.4101, -237.1162) knots 0 0 0 1 2 2 2
  spline S219 degree 2 poles (-1.4101, -237.1162) (-0.8815, -236.9521) (-0.3164, -236.3779) (-0.2252, -235.9131) knots 0 0 0 1 2 2 2
  line L144 (5.3803, -246.2216) -> (-3.6614, -246.2216)
  spline S220 degree 2 poles (-3.6614, -246.2216) (-3.9622, -246.2216) (-4.0898, -246.3584) knots 0 0 0 1 1 1
  spline S221 degree 2 poles (-4.0898, -246.3584) (-4.1627, -246.4313) (-4.2083, -246.568) (-4.2812, -246.9235) knots 0 0 0 1 2 2 2
  spline S222 degree 2 poles (-4.2812, -246.9235) (-4.3632, -247.3701) (-4.7005, -247.3701) knots 0 0 0 1 1 1
  spline S223 degree 2 poles (-4.7005, -247.3701) (-4.901, -247.3701) (-5.0286, -247.1331) knots 0 0 0 1 1 1
  spline S224 degree 2 poles (-5.0286, -247.1331) (-5.1197, -246.9508) (-5.1197, -246.5498) knots 0 0 0 1 1 1
  line L145 (-5.1197, -246.5498) -> (-5.1197, -246.2308)
  line L146 (-5.1197, -246.2308) -> (-5.1197, -242.1201)
  line L147 (-5.1197, -242.1201) -> (-5.1197, -241.8831)
  spline S225 degree 2 poles (-5.1197, -241.8831) (-5.1197, -241.5459) (-4.9101, -241.1904) (-4.7187, -241.1904) knots 0 0 0 1 2 2 2
  spline S226 degree 2 poles (-4.7187, -241.1904) (-4.4088, -241.1904) (-4.3085, -241.555) knots 0 0 0 1 1 1
  spline S227 degree 2 poles (-4.3085, -241.555) (-4.2174, -241.8649) (-4.1809, -241.9651) (-4.108, -242.0198) knots 0 0 0 1 2 2 2
  spline S228 degree 2 poles (-4.108, -242.0198) (-3.9895, -242.1292) (-3.7161, -242.1292) knots 0 0 0 1 1 1
  line L148 (-3.7161, -242.1292) -> (3.9766, -242.1292)
  spline S229 degree 2 poles (3.9766, -242.1292) (4.25, -242.1292) (4.3685, -242.0198) knots 0 0 0 1 1 1
  spline S230 degree 2 poles (4.3685, -242.0198) (4.4415, -241.9651) (4.4779, -241.8649) (4.5599, -241.555) knots 0 0 0 1 2 2 2
  spline S231 degree 2 poles (4.5599, -241.555) (4.6602, -241.1904) (4.9792, -241.1904) knots 0 0 0 1 1 1
  spline S232 degree 2 poles (4.9792, -241.1904) (5.1706, -241.1904) (5.3803, -241.5459) (5.3803, -241.8831) knots 0 0 0 1 2 2 2
  line L149 (5.3803, -241.8831) -> (5.3803, -242.1201)
  line L150 (5.3803, -242.1201) -> (5.3803, -246.2216)
  spline S233 degree 2 poles (0.0209, -249.0563) (-0.0794, -249.9039) (-0.3437, -250.8245) (-0.5716, -251.1891) knots 0 0 0 1 2 2 2
  spline S234 degree 2 poles (-0.5716, -251.1891) (-0.8085, -251.5719) (-1.4648, -251.9912) (-1.8385, -251.9912) knots 0 0 0 1 2 2 2
  line L151 (-1.8385, -251.9912) -> (-3.4244, -251.9912)
  spline S235 degree 2 poles (-3.4244, -251.9912) (-3.6796, -251.9912) (-3.6796, -252.1826) knots 0 0 0 1 1 1
  spline S236 degree 2 poles (-3.6796, -252.1826) (-3.6796, -252.2555) (-3.6067, -252.3649) (-3.5065, -252.456) knots 0 0 0 1 2 2 2
  spline S237 degree 2 poles (-3.5065, -252.456) (-3.2421, -252.6839) (-3.2421, -252.9209) knots 0 0 0 1 1 1
  spline S238 degree 2 poles (-3.2421, -252.9209) (-3.2421, -253.0849) (-3.5156, -253.3948) (-3.6614, -253.3948) knots 0 0 0 1 2 2 2
  spline S239 degree 2 poles (-3.6614, -253.3948) (-3.8984, -253.3948) (-4.582, -252.8479) (-4.8554, -252.4469) knots 0 0 0 1 2 2 2
  spline S240 degree 2 poles (-4.8554, -252.4469) (-5.1015, -252.0641) (-5.3294, -251.18) (-5.3294, -250.5784) knots 0 0 0 1 2 2 2
  spline S241 degree 2 poles (-5.3294, -250.5784) (-5.3294, -249.3662) (-4.1627, -247.999) (-3.1328, -247.999) knots 0 0 0 1 2 2 2
  line L152 (-3.1328, -247.999) -> (-1.8385, -247.999)
  spline S242 degree 2 poles (-1.8385, -247.999) (-1.4101, -247.999) (-1.3372, -247.9899) knots 0 0 0 1 1 1
  spline S243 degree 2 poles (-1.3372, -247.9899) (-1.0273, -247.9443) (-0.8085, -247.7347) knots 0 0 0 1 1 1
  spline S244 degree 2 poles (-0.8085, -247.7347) (-0.5351, -247.4612) (-0.4895, -246.969) knots 0 0 0 1 1 1
  line L153 (-0.4895, -246.969) -> (0.3308, -246.969)
  spline S245 degree 2 poles (0.3308, -246.969) (0.3946, -247.4612) (0.5495, -247.68) knots 0 0 0 1 1 1
  spline S246 degree 2 poles (0.5495, -247.68) (0.6862, -247.8623) (1.0417, -247.999) (1.3881, -247.999) knots 0 0 0 1 2 2 2
  line L154 (1.3881, -247.999) -> (3.4297, -247.999)
  spline S247 degree 2 poles (3.4297, -247.999) (3.9128, -247.999) (4.3868, -247.5433) (4.5235, -246.9599) knots 0 0 0 1 2 2 2
  line L155 (4.5235, -246.9599) -> (5.3803, -246.9599)
  line L156 (5.3803, -246.9599) -> (5.3803, -247.1969)
  spline S248 degree 2 poles (5.3803, -247.1969) (5.3803, -248.2177) (5.3165, -248.9378) knots 0 0 0 1 1 1
  spline S249 degree 2 poles (5.3165, -248.9378) (5.2344, -250.0042) (4.7331, -250.8427) knots 0 0 0 1 1 1
  spline S250 degree 2 poles (4.7331, -250.8427) (4.0222, -252.055) (2.6915, -252.055) knots 0 0 0 1 1 1
  spline S251 degree 2 poles (2.6915, -252.055) (1.6068, -252.055) (0.9141, -251.2438) knots 0 0 0 1 1 1
  spline S252 degree 2 poles (0.9141, -251.2438) (0.6224, -250.9065) (0.2579, -249.986) (0.0209, -249.0563) knots 0 0 0 1 2 2 2
  point P0 (0, 0)
  constraints: 2 other
extrude "Extrusion3" cut sketch "Skizze8" against normal blind 10
equation "\"d125\" = Stärke"
equation "\"d6\" = Stärke"
equation "\"d7\" = BreiteBiegungsfreistellung"
equation "\"d8\" = TiefeBiegungsfreistellung"
equation "\"d9\" = MinimalRest"
equation "\"d10\" = Übergangsradius"
equation "\"d13\" = Biegeradius"
equation "\"d14\" = GrößeEckenfreistellung"
equation "\"d15\" = Abstandsgröße"
equation "\"d16\" = JacobiRadiusGröße"
equation "\"d17\" = BreiteBiegungsfreistellung"
equation "\"d18\" = TiefeBiegungsfreistellung"
equation "\"d19\" = MinimalRest"
equation "\"d20\" = Übergangsradius"
equation "\"d23\" = Biegeradius"
equation "\"d24\" = GrößeEckenfreistellung"
equation "\"d25\" = Abstandsgröße"
equation "\"d26\" = JacobiRadiusGröße"
equation "\"Biegeradius\" = Stärke"
equation "\"BreiteBiegungsfreistellung\" = Stärke"
equation "\"TiefeBiegungsfreistellung\" = 0.5 * Stärke"
equation "\"GrößeEckenfreistellung\" = 4 * Stärke"
equation "\"MinimalRest\" = 2 * Stärke"
equation "\"Übergangsradius\" = Biegeradius"
equation "\"JacobiRadiusGröße\" = Biegeradius"
equation "\"Abstandsgröße\" = Stärke"
equation "\"Stärke\" = 2"
